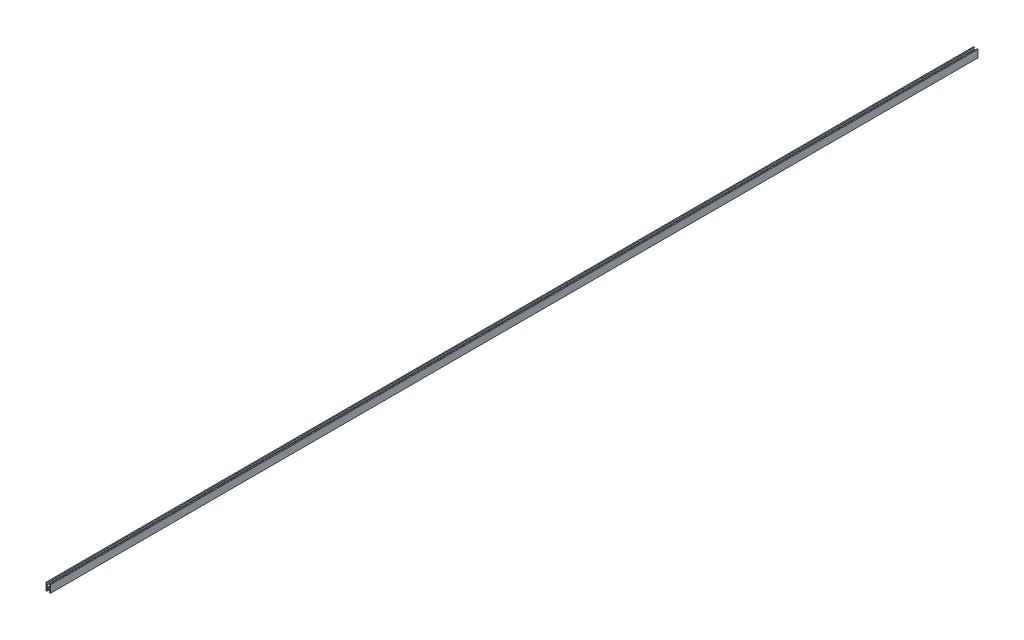
# Autodesk Inventor part: SP40-04B TRAVESAÑO CENTRAL
Saved by Autodesk Inventor 2025 (Build 290162000, 162)
## iProperties
Created: 2026-01-20
Part Number: SP40-04B TRAVESAÑO CENTRAL
Material: Aluminio
Document SubType Name: Modeling
Designer: ROLANDO
Density: 2.7 g/cm^3
Appearance: Satinado
Author: ROLANDO
Autodesk Inventor part; units mm, degrees
ref_plane "YZ Plane" through (0, 0, 0) normal (1, 0, 0) x (0, 1, 0)
ref_plane "XZ Plane" through (0, 0, 0) normal (0, 1, 0) x (-1, 0, 0)
ref_plane "XY Plane" through (0, 0, 0) normal (0, 0, 1) x (1, 0, 0)
sketch "Boceto1" plane through (0, 0, 0) normal (0, 0, 1) x (1, 0, 0)
  line L0 (-4.7609, 3.4664) -> (-4.7609, -16.5336)
  line L1 (-4.7609, -16.5336) -> (0.4391, -16.5336)
  line L2 (0.4391, -16.5336) -> (0.4391, -14.8936)
  line L3 (-0.9609, -15.1336) -> (-3.3609, -15.1336)
  line L4 (-3.3609, -15.1336) -> (-3.3609, -3.0336)
  line L5 (-2.8609, -2.5336) -> (17.5391, -2.5336)
  line L6 (18.0391, -3.0336) -> (18.0391, -7.2336)
  line L7 (18.0391, -7.2336) -> (14.2391, -7.2336)
  line L8 (14.2391, -7.2336) -> (14.2391, -8.8736)
  line L9 (14.9333, -9.8836) -> (15.6391, -9.8836)
  line L10 (15.6391, -9.8836) -> (15.6391, -8.6336)
  line L11 (15.6391, -8.6336) -> (18.0391, -8.6336)
  line L12 (18.0391, -8.6336) -> (18.0391, -15.1336)
  line L13 (18.0391, -15.1336) -> (15.6391, -15.1336)
  line L14 (15.6391, -15.1336) -> (15.6391, -13.8836)
  line L15 (15.6391, -13.8836) -> (14.9333, -13.8836)
  line L16 (14.2391, -14.8936) -> (14.2391, -16.5336)
  line L17 (14.2391, -16.5336) -> (19.4391, -16.5336)
  line L18 (19.4391, -16.5336) -> (19.4391, 3.4664)
  line L19 (-3.3609, 3.4664) -> (-3.3609, -0.6336)
  line L20 (18.0391, -0.6336) -> (18.0391, 3.4664)
  line L21 (7.3391, 9.4664) -> (7.3391, -1.1336) construction
  line L22 (-2.8609, -1.1336) -> (17.5391, -1.1336)
  line L23 (-0.9609, -15.1336) -> (-0.9609, -13.8836)
  line L24 (-0.9609, -13.8836) -> (-0.2551, -13.8836)
  line L25 (-0.2551, -13.8836) -> (0.4391, -14.8936)
  line L26 (14.2391, -8.8736) -> (14.9333, -9.8836)
  line L27 (14.2391, -14.8936) -> (14.9333, -13.8836)
  arc A0 (-2.8609, -2.5336) -> (-3.3609, -3.0336) centre (-2.8609, -3.0336) ccw
  arc A1 (-3.3609, -0.6336) -> (-2.8609, -1.1336) centre (-2.8609, -0.6336) ccw
  arc A2 (17.5391, -1.1336) -> (18.0391, -0.6336) centre (17.5391, -0.6336) ccw
  arc A3 (18.0391, -3.0336) -> (17.5391, -2.5336) centre (17.5391, -3.0336) ccw
  line L28 (-4.7609, 3.4664) -> (-4.7609, 23.4664)
  line L29 (-4.7609, 23.4664) -> (0.4391, 23.4664)
  line L30 (0.4391, 23.4664) -> (0.4391, 21.8264)
  line L31 (-0.9609, 22.0664) -> (-3.3609, 22.0664)
  line L32 (-3.3609, 22.0664) -> (-3.3609, 9.9664)
  line L33 (-2.8609, 9.4664) -> (17.5391, 9.4664)
  line L34 (18.0391, 9.9664) -> (18.0391, 14.1664)
  line L35 (18.0391, 14.1664) -> (14.2391, 14.1664)
  line L36 (14.2391, 14.1664) -> (14.2391, 15.8064)
  line L37 (14.9333, 16.8164) -> (15.6391, 16.8164)
  line L38 (15.6391, 16.8164) -> (15.6391, 15.5664)
  line L39 (15.6391, 15.5664) -> (18.0391, 15.5664)
  line L40 (18.0391, 15.5664) -> (18.0391, 22.0664)
  line L41 (18.0391, 22.0664) -> (15.6391, 22.0664)
  line L42 (15.6391, 22.0664) -> (15.6391, 20.8164)
  line L43 (15.6391, 20.8164) -> (14.9333, 20.8164)
  line L44 (14.2391, 21.8264) -> (14.2391, 23.4664)
  line L45 (14.2391, 23.4664) -> (19.4391, 23.4664)
  line L46 (19.4391, 23.4664) -> (19.4391, 3.4664)
  line L47 (-3.3609, 3.4664) -> (-3.3609, 7.5664)
  line L48 (18.0391, 7.5664) -> (18.0391, 3.4664)
  line L49 (7.3391, -1.1336) -> (7.3391, 9.4664) construction
  arc A4 (8.4391, 3.5111) -> (6.2391, 3.5111) centre (7.3391, 5.4164) ccw
  line L50 (4.9522, 5.6664) -> (5.1534, 5.6664)
  line L51 (4.9522, 5.1664) -> (5.1534, 5.1664)
  line L52 (-2.8609, 8.0664) -> (3.8304, 8.0664)
  line L53 (10.8478, 8.0664) -> (17.5391, 8.0664)
  line L54 (4.0797, 5.4164) -> (9.7739, 5.4164) construction
  line L55 (9.726, 5.6664) -> (9.5249, 5.6664)
  line L56 (9.726, 5.1664) -> (9.5249, 5.1664)
  line L57 (7.5891, 7.8033) -> (7.5891, 7.6021)
  line L58 (7.0891, 7.8033) -> (7.0891, 7.6021)
  arc A5 (7.5891, 7.8033) -> (7.0891, 7.8033) centre (7.3391, 5.4164) ccw
  arc A6 (9.726, 5.1664) -> (9.726, 5.6664) centre (7.3391, 5.4164) ccw
  arc A7 (4.9522, 5.6664) -> (4.9522, 5.1664) centre (7.3391, 5.4164) ccw
  circle A8 centre (7.3391, 5.4164) radius 2.4 construction
  line L59 (6.2391, 1.9728) -> (6.2391, 3.5111)
  line L60 (8.4391, 1.9728) -> (8.4391, 3.5111)
  arc A9 (8.4391, 1.9728) -> (10.4214, 7.3051) centre (7.3391, 5.4164) ccw
  arc A10 (4.2568, 7.3051) -> (6.2391, 1.9728) centre (7.3391, 5.4164) ccw
  line L61 (-0.9609, 22.0664) -> (-0.9609, 20.8164)
  line L62 (-0.9609, 20.8164) -> (-0.2551, 20.8164)
  line L63 (-0.2551, 20.8164) -> (0.4391, 21.8264)
  line L64 (14.2391, 15.8064) -> (14.9333, 16.8164)
  line L65 (14.2391, 21.8264) -> (14.9333, 20.8164)
  arc A11 (-3.3609, 9.9664) -> (-2.8609, 9.4664) centre (-2.8609, 9.9664) ccw
  arc A12 (-2.8609, 8.0664) -> (-3.3609, 7.5664) centre (-2.8609, 7.5664) ccw
  arc A13 (18.0391, 7.5664) -> (17.5391, 8.0664) centre (17.5391, 7.5664) ccw
  arc A14 (17.5391, 9.4664) -> (18.0391, 9.9664) centre (17.5391, 9.9664) ccw
  arc A15 (4.2568, 7.3051) -> (3.8304, 8.0664) centre (3.8304, 7.5664) ccw
  arc A16 (10.8478, 8.0664) -> (10.4214, 7.3051) centre (10.8478, 7.5664) ccw
  point P0 (18.0391, -11.8836)
  point P1 (4.8803, 8.0664)
  point P2 (9.7979, 8.0664)
  point P3 (18.0391, 18.8164)
  dimension "d0" = 1.4
  dimension "d1" = 1.4
  dimension "d2" = 1.4
  dimension "d3" = 1.4
  dimension "d4" = 1.4
  dimension "d5" = 1.4
  dimension "d6" = 1.4
  dimension "d7" = 1.4
  dimension "d8" = 1.4
  dimension "d9" = 1.4
  dimension "d43" = 14
  dimension "d44" = 4
  dimension "d45" = 9.3
  dimension "d46" = 6.5
  dimension "d47" = 24.2
  dimension "d48" = 5.2
  dimension "d49" = 1.4
  dimension "d50" = 5.2
  dimension "d51" = 13.8
  dimension "d52" = 21.4
  dimension "d63" = 2.65
  dimension "d64" = 1.64
  dimension "d65" = 34.5
  dimension "d66" = 2
  dimension "d67" = 2
  dimension "d68" = 2.4
  dimension "d69" = 3.01
  dimension "d70" = 6.02
  dimension "d71" = 34.5
  dimension "d72" = 111
  dimension "d74" = 0.7058
  dimension "d75" = 0.7058
  dimension "d86" = 0.5
  dimension "d87" = 0.5
  dimension "d88" = 40
  dimension "d89" = 1.4
  dimension "d90" = 9.2
  dimension "d91" = 26
  dimension "d92" = 4.05
  dimension "d93" = 3.615
  dimension "d94" = 3.615
  dimension "d95" = 2.4
  dimension "d96" = 2.4
  dimension "d97" = 2.4
  dimension "d98" = 4.8
  dimension "d99" = 2.2
  dimension "d100" = 90
  dimension "d101" = 90
  dimension "d102" = 90
  dimension "d103" = 90
  dimension "d104" = 90
  dimension "d105" = 90
  dimension "d106" = 90
  dimension "d107" = 90
  dimension "d108" = 90
  dimension "d109" = 90
  dimension "d110" = 3.8
  dimension "d111" = 5.2
  dimension "d112" = 11
  dimension "d113" = 11.85
  dimension "d114" = 12.1
  dimension "d115" = 12.35
  dimension "d116" = 13.2
  dimension "d117" = 19
  constraints: 132 end point, 40 point on circle, 24 tangent, 22 parallel, 17 centre point, 17 perpendicular, 8 equal radius, 6 point on line, 6 vertical, 5 collinear, 3 coincident, 3 midpoint, 1 horizontal
  measures "d0" distance between parallel lines of L19 L0
  measures "d1" distance between parallel lines of L0 L4
  measures "d2" distance between parallel lines of L1 L3
  measures "d3" distance between parallel lines of L18 L20
  measures "d4" distance between parallel lines of L18 L6
  measures "d5" distance between parallel lines of L18 L12
  measures "d6" distance between parallel lines of L17 L13
  measures "d7" distance between parallel lines of L7 L11
  measures "d8" distance between parallel lines of L8 L10
  measures "d9" distance between parallel lines of L16 L14
  measures "d43" distance between parallel lines of L17 L5
  measures "d44" distance between parallel lines of L15 L9
  measures "d45" distance between parallel lines of L17 L7
  measures "d46" distance between parallel lines of L13 L11
  measures "d47" distance between parallel lines of L18 L0
  measures "d48" distance between parallel lines of L0 L2
  measures "d49" distance between parallel lines of L2 L23
  measures "d50" distance between parallel lines of L18 L16
  measures "d51" distance between parallel lines of L2 L16
  measures "d52" distance between parallel lines of L12 L4
  measures "d63" distance between parallel lines of L24 L1
  measures "d64" distance of L1.end L2.end
  measures "d65" angle of L2 L25
  measures "d66" distance from line of point (18.039, -11.884) L9
  measures "d67" distance from line of point (18.039, -11.884) L15
  measures "d68" distance between parallel lines of L12 L10
  measures "d69" vertical distance of point (18.039, -11.884) L8.end
  measures "d70" distance of L8.end L16.start
  measures "d71" angle of L10 L26
  measures "d72" angle of L27 L26
  measures "d74" distance of L9.start L9.end
  measures "d75" distance of L14.end L15.end
  measures "d86" radius of A0
  measures "d87" radius of A1
  measures "d88" distance between parallel lines of L17 L45
  measures "d89" distance between parallel lines of L5 L22
  measures "d90" distance between parallel lines of L22 L53
  measures "d91" distance between parallel lines of L17 L33
  measures "d92" distance from line of L33 A10.centre
  measures "d93" radius of A10
  measures "d94" radius of A9
  measures "d95" radius of A7
  measures "d96" radius of A6
  measures "d97" radius of A5
  measures "d98" diameter of A8
  measures "d99" radius of A4
  measures "d100" angle of L43 L18
  measures "d101" angle of L41 L18
  measures "d102" angle of L55 L18
  measures "d103" angle of L56 L18
  measures "d104" angle of L46 L52
  measures "d105" angle of L43 L48
  measures "d106" angle of L43 L40
  measures "d107" angle of L43 L42
  measures "d108" angle of L44 L43
  measures "d109" angle of L43 L47
  measures "d110" distance between parallel lines of L38 L18
  measures "d111" distance between parallel lines of L36 L18
  measures "d112" distance between parallel lines of L60 L18
  measures "d113" distance between parallel lines of L57 L18
  measures "d114" distance between parallel lines of L18 L49
  measures "d115" distance between parallel lines of L58 L18
  measures "d116" distance between parallel lines of L59 L18
  measures "d117" distance between parallel lines of L30 L18
extrude "Extrusión1" add sketch "Boceto1" against normal blind 5000
